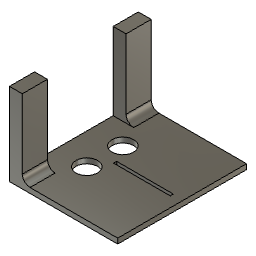
Slit_1-2mm (Autodesk Fusion 360 design; units mm, degrees)
Autodesk Fusion 360 part; units mm, degrees
sketch "Sketch1" plane through (0, 0, 0) normal (0, 0, 1) x (1, 0, 0)
  line L0 (21, -25) -> (-21, -25)
  line L1 (-21, -25) -> (-21, 25)
  line L2 (-21, 25) -> (21, 25)
  line L3 (21, 25) -> (21, -25)
  line L4 (21, -25) -> (-21, 25) construction
  line L5 (-21, -25) -> (21, 25) construction
  line L6 (-21, 0) -> (-9, 0) construction
  line L7 (-9, 0) -> (-9, -7) construction
  line L8 (-9, -7) -> (-21, -7) construction
  line L9 (-21, -7) -> (-21, 0) construction
  line L10 (-21, 0) -> (-9, 0) construction
  line L11 (-9, 0) -> (-9, 7) construction
  line L12 (-9, 7) -> (-21, 7) construction
  line L13 (-21, 7) -> (-21, 0) construction
  circle A0 centre (-9, 7) radius 4.2
  circle A1 centre (-9, -7) radius 4.2
  line L14 (-21, 0) -> (6, 0) construction
  line L15 (17, -0.6) -> (-5, -0.6)
  line L16 (-5, -0.6) -> (-5, 0.6)
  line L17 (-5, 0.6) -> (17, 0.6)
  line L18 (17, 0.6) -> (17, -0.6)
  line L19 (17, -0.6) -> (-5, 0.6) construction
  line L20 (-5, -0.6) -> (17, 0.6) construction
  point P0 (6, 0)
  dimension "d1" = 42
  dimension "d2" = 50
  dimension "d3" = 12
  dimension "d4" = 7
  dimension "d5" = 12
  dimension "d6" = 7
  dimension "d7" = 8.4
  dimension "d8" = 8.4
  dimension "d9" = 27
  dimension "d10" = 22
  dimension "d11" = 1.2
  constraint horizontal L0
  constraint perpendicular L0 L1
  constraint parallel L0 L2
  constraint parallel L1 L3
  constraint coincident L4 origin
  constraint coincident L5 origin
  constraint horizontal L6
  constraint vertical L7
  constraint horizontal L8
  constraint vertical L9
  constraint midpoint L1 L6.start
  constraint horizontal L10
  constraint vertical L11
  constraint horizontal L12
  constraint vertical L13
  constraint coincident L11.end L12.start
  constraint coincident L7.end L8.start
  constraint perpendicular L9 L14
  constraint horizontal L15
  constraint perpendicular L15 L16
  constraint parallel L15 L17
  constraint parallel L16 L18
  constraint coincident L19 P0
  constraint coincident L20 P0
  constraint coincident P0 L14.end
  measures "d1" distance of L1.end L2.end
  measures "d2" distance of L0.end L1.end
  measures "d3" distance of L6.start L6.end
  measures "d4" distance of L6.start L8.end
  measures "d5" distance of L6.start L6.end
  measures "d6" distance of L6.start L12.end
  measures "d7" diameter of A0
  measures "d8" diameter of A1
  measures "d9" distance of L6.start P0
  measures "d10" distance of L16.end L17.end
  measures "d11" distance of L15.end L16.end
extrude "Extrude1" add sketch "Sketch1" along normal blind 2 makes body 1
sketch "Sketch2" plane through (0, 0, 2) normal (0, 0, 1) x (-1, 0, 0)
  line L0 (5, -0.6) -> (-17, -0.6)
  line L1 (-17, -0.6) -> (-17, 0.6)
  line L2 (-17, 0.6) -> (5, 0.6)
  line L3 (5, 0.6) -> (5, -0.6)
  circle A0 centre (9, 7) radius 4.2
  circle A1 centre (9, -7) radius 4.2
  line L4 (-21, -25) -> (21, -25)
  line L5 (21, -25) -> (21, 25)
  line L6 (21, 25) -> (-21, 25)
  line L7 (-21, 25) -> (-21, -25)
  line L8 (21, -25) -> (16, -25)
  line L9 (16, -25) -> (16, -15.25)
  line L10 (16, -15.25) -> (21, -15.25)
  line L11 (21, -15.25) -> (21, -25)
  line L12 (21, 25) -> (16, 25)
  line L13 (16, 25) -> (16, 15.25)
  line L14 (16, 15.25) -> (21, 15.25)
  line L15 (21, 15.25) -> (21, 25)
  dimension "d14" = 5
  dimension "d15" = 9.75
  dimension "d16" = 5
  dimension "d17" = 9.75
  constraint horizontal L8
  constraint vertical L9
  constraint horizontal L10
  constraint vertical L11
  constraint coincident L4.end L5.start
  constraint horizontal L12
  constraint vertical L13
  constraint horizontal L14
  constraint vertical L15
  constraint coincident L5.end L6.start
  measures "d14" distance of L4.end L8.end
  measures "d15" distance of L4.end L10.end
  measures "d16" distance of L5.end L12.end
  measures "d17" distance of L5.end L14.end
extrude "Extrude2" add sketch "Sketch2" along normal blind 30 contours L4 L5 L8 L9 L10 L11 | L5 L6 L12 L13 L14 L15 bodies 1
fillet "Fillet1" radius 3 2 edges at (-16, -20.125, 2) (-16, 20.125, 2) on bodies 1
copy_body "Body->Comp1" bodies 1 removing the originals makes body 2 in component "Slit"
component "Slit" placed x (1, 0, 0) y (0, 1, 0) z (0, 0, 1) at (0, 0, 0)
